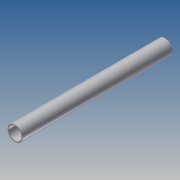
# Autodesk Inventor part: 2p5vss
Saved by Autodesk Inventor 2014 SP1 (Build 180222100, 222)
## iProperties
Company: HERA Project
Created: 2013-06-11
Part Number: 2p5vss
Material: PVC-Piping
Document SubType Name: Modeling
Designer: David DeBoer
Density: 1.4 g/cm^3
Description: support vertical spar
Mass: 468.384 g
Surface Area: 1724.47 cm^2
Volume: 334.56 cm^3
Appearance: Smooth - White
Author: David DeBoer
Title: Hub-supporthold
Autodesk Inventor part; units mm, degrees
ref_plane "YZ Plane" through (0, 0, 0) normal (1, 0, 0) x (0, 1, 0)
ref_plane "XZ Plane" through (0, 0, 0) normal (0, 1, 0) x (-1, 0, 0)
ref_plane "XY Plane" through (0, 0, 0) normal (0, 0, 1) x (1, 0, 0)
sketch "Sketch1" plane through (0, 0, 0) normal (0, 0, 1) x (1, 0, 0)
  circle A0 centre (0, 0) radius 30.1625
  circle A1 centre (0, 0) radius 26.2509
  dimension "d0" = 60.325
  dimension "d2" = 3.9116
  constraints: 2 centre point, 1 coincident
  measures "d0" diameter of A0
  measures "d2" radial gap between concentric circles of A1 A0
extrude "Extrusion1" add sketch "Sketch1" along normal blind 604.52
body "Solid1"
